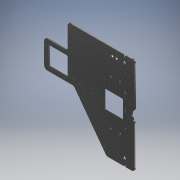
# Autodesk Inventor part: CAR SIDE PLATE I
Saved by Autodesk Inventor 2017 (Build 210142000, 142)
## iProperties
Part Number: CAR SIDE PLATE I
Material: Genérico
Document SubType Name: Modeling
Designer: Cristian
Density: 1 g/cm^3
Appearance: Valor por defecto
Author: Cristian
Autodesk Inventor part; units mm, degrees
ref_plane "YZ Plane" through (0, 0, 0) normal (1, 0, 0) x (0, 1, 0)
ref_plane "XZ Plane" through (0, 0, 0) normal (0, 1, 0) x (-1, 0, 0)
ref_plane "XY Plane" through (0, 0, 0) normal (0, 0, 1) x (1, 0, 0)
sketch "Boceto1" plane through (0, 0, 0) normal (0, 1, 0) x (-1, 0, 0)
  line L0 (0, 0) -> (273.05, 0)
  line L1 (273.05, 0) -> (273.05, -101.6)
  line L2 (273.05, -101.6) -> (368.3, -101.6)
  line L3 (368.3, -101.6) -> (368.3, -212.725)
  line L4 (0, 0) -> (0, -393.7)
  line L5 (0, -393.7) -> (114.3, -393.7)
  line L6 (368.3, -212.725) -> (247.65, -212.725)
  line L7 (247.65, -212.725) -> (114.3, -393.7)
  dimension "d0" = 273.05
  dimension "d1" = 101.6
  dimension "d2" = 95.25
  dimension "d3" = 111.125
  dimension "d4" = 393.7
  dimension "d50" = 114.3
  dimension "d51" = 133.35
  constraints: 16 end point, 3 horizontal, 2 perpendicular, 2 vertical
  measures "d0" distance of L0.start L0.end
  measures "d1" distance of L0.end L1.end
  measures "d2" distance of L1.end L2.end
  measures "d3" distance of L2.end L3.end
  measures "d4" distance of L0.start L4.end
  measures "d50" distance of L4.end L5.end
  measures "d51" horizontal distance of L5.end L6.end
extrude "Extrusión1" add sketch "Boceto1" along normal blind 5
fillet "Empalme1" radius 12.7 7 edges at (-368.3, 2.5, -101.6) (-273.05, 2.5, 0) (-368.3, 2.5, -212.725) (-247.65, 2.5, -212.725) (-114.3, 2.5, -393.7) (0, 2.5, -393.7) (0, 2.5, 0)
fillet "Empalme2" radius 6.35 1 edges at (-273.05, 2.5, -101.6)
sketch "Boceto2" plane through (0, 5, 0) normal (0, 1, 0) x (1, 0, 0)
  line L0 (-349.25, 119.0625) -> (-273.05, 119.0625)
  line L1 (-273.05, 119.0625) -> (-273.05, 195.2625)
  line L2 (-273.05, 195.2625) -> (-349.25, 195.2625)
  line L3 (-349.25, 195.2625) -> (-349.25, 119.0625)
  line L4 (-368.3, 200.025) -> (-368.3, 114.3) projected
  line L5 (-254.0674, 212.725) -> (-355.6, 212.725) projected
  line L6 (-355.6, 101.6) -> (-279.4, 101.6) projected
  line L7 (-260.35, 0) -> (-12.7, 0) projected
  line L8 (-43.6563, 0) -> (-38.1, 0)
  line L9 (-38.1, 0) -> (-38.1, 6.35)
  line L10 (-38.1, 6.35) -> (-43.6562, 6.35)
  line L11 (-43.6562, 6.35) -> (-43.6563, 0)
  line L12 (-12.7, 393.7) -> (-107.8826, 393.7) projected
  line L13 (0, 12.7) -> (0, 381) projected
  circle A0 centre (-98.0281, 104.775) radius 4.3656
  circle A1 centre (-59.9281, 104.775) radius 4.3656
  circle A2 centre (-98.0281, 288.925) radius 4.3656
  circle A3 centre (-59.9281, 288.925) radius 4.3656
  line L14 (-123.825, 158.75) -> (-47.625, 158.75)
  line L15 (-47.625, 158.75) -> (-47.625, 234.95)
  line L16 (-47.625, 234.95) -> (-123.825, 234.95)
  line L17 (-123.825, 234.95) -> (-123.825, 158.75)
  circle A4 centre (-42.6641, 365.125) radius 6.35
  circle A5 centre (-42.6641, 28.575) radius 6.35
  line L18 (-107.8826, 393.7) -> (-12.7, 393.7) projected
  line L19 (-43.6563, 393.7) -> (-38.1, 393.7)
  line L20 (-38.1, 393.7) -> (-38.1, 387.35)
  line L21 (-38.1, 387.35) -> (-43.6563, 387.35)
  line L22 (-43.6563, 387.35) -> (-43.6563, 393.7)
  line L23 (-43.6563, 127) -> (-38.1, 127)
  line L24 (-38.1, 127) -> (-38.1, 140.0969)
  line L25 (-38.1, 140.0969) -> (-43.6563, 140.0969)
  line L26 (-43.6563, 140.0969) -> (-43.6563, 127)
  line L27 (-43.6563, 190.5) -> (-38.1, 190.5)
  line L28 (-38.1, 190.5) -> (-38.1, 203.5969)
  line L29 (-38.1, 203.5969) -> (-43.6563, 203.5969)
  line L30 (-43.6563, 203.5969) -> (-43.6563, 190.5)
  line L31 (-43.6563, 254) -> (-38.1, 254)
  line L32 (-38.1, 254) -> (-38.1, 267.0969)
  line L33 (-38.1, 267.0969) -> (-43.6563, 267.0969)
  line L34 (-43.6563, 267.0969) -> (-43.6563, 254)
  circle A6 centre (-73.025, 29.3688) radius 3.9687
  circle A7 centre (-90.4875, 29.3688) radius 3.9688
  point P0 (0, 0)
  dimension "d11" = 76.2
  dimension "d17" = 17.4625
  dimension "d18" = 19.05
  dimension "d19" = 76.2
  dimension "d20" = 5.5563
  dimension "d22" = 6.35
  dimension "d24" = 38.1
  dimension "d27" = 8.7312
  dimension "d38" = 76.2
  dimension "d39" = 76.2
  dimension "d40" = 158.75
  dimension "d42" = 12.7
  dimension "d43" = 28.575
  dimension "d44" = 42.6641
  dimension "d47" = 12.7
  dimension "d52" = 38.1
  dimension "d53" = 5.5563
  dimension "d54" = 6.35
  dimension "d55" = 47.625
  dimension "d56" = 8.7312
  dimension "d57" = 98.0281
  dimension "d58" = 38.1
  dimension "d59" = 53.975
  dimension "d60" = 53.975
  dimension "d61" = 184.15
  dimension "d62" = 184.15
  dimension "d63" = 38.1
  dimension "d64" = 8.7312
  dimension "d65" = 8.7312
  dimension "d66" = 98.0281
  dimension "d67" = 42.6641
  dimension "d68" = 28.575
  dimension "d69" = 5.5563
  dimension "d70" = 5.5563
  dimension "d71" = 5.5563
  dimension "d72" = 13.0969
  dimension "d73" = 13.0969
  dimension "d74" = 13.0969
  dimension "d75" = 38.1
  dimension "d80" = 63.5
  dimension "d81" = 63.5
  dimension "d82" = 127
  dimension "d92" = 7.9375
  dimension "d93" = 7.9375
  dimension "d94" = 25.4
  dimension "d96" = 25.4
  dimension "d97" = 25.4
  dimension "d98" = 25.4
  constraints: 56 end point, 14 parallel, 8 centre point, 7 horizontal, 7 perpendicular, 3 point on line, 1 collinear
  measures "d11" distance of L2.end L0.start
  measures "d17" distance between parallel lines of L0 L6
  measures "d18" distance between parallel lines of L3 L4
  measures "d19" distance of L1.end L2.end
  measures "d20" distance between parallel lines of L9 L11
  measures "d22" distance of L10.end L8.start
  measures "d24" distance between parallel lines of L13 L9
  measures "d27" diameter of A1
  measures "d38" distance of L16.end L14.start
  measures "d39" distance between parallel lines of L15 L17
  measures "d40" distance between parallel lines of L7 L14
  measures "d42" diameter of A4
  measures "d43" distance from line of L12 A4.centre
  measures "d44" distance from line of L13 A4.centre
  measures "d47" diameter of A5
  measures "d52" distance between parallel lines of L13 L20
  measures "d53" distance between parallel lines of L20 L22
  measures "d54" distance of L21.end L19.start
  measures "d55" distance between parallel lines of L13 L15
  measures "d56" diameter of A0
  measures "d57" distance from line of L13 A0.centre
  measures "d58" distance of A1.centre A0.centre
  measures "d59" distance from line of L14 A0.centre
  measures "d60" distance from line of L14 A1.centre
  measures "d61" distance of A2.centre A0.centre
  measures "d62" distance of A1.centre A3.centre
  measures "d63" distance of A3.centre A2.centre
  measures "d64" diameter of A2
  measures "d65" diameter of A3
  measures "d66" distance from line of L13 A2.centre
  measures "d67" distance from line of L13 A5.centre
  measures "d68" distance from line of L7 A5.centre
  measures "d69" distance of L25.end L24.end
  measures "d70" distance of L29.end L28.end
  measures "d71" distance between parallel lines of L32 L34
  measures "d72" distance between parallel lines of L25 L23
  measures "d73" distance of L27.end L28.end
  measures "d74" distance of L31.end L32.end
  measures "d75" distance between parallel lines of L13 L24
  measures "d80" distance between parallel lines of L27 L23
  measures "d81" distance between parallel lines of L31 L27
  measures "d82" distance between parallel lines of L7 L23
  measures "d92" diameter of A6
  measures "d93" diameter of A7
  measures "d94" distance edge to line of A6 L11
  measures "d96" distance edge to line of A6 L7
  measures "d97" distance edge to line of A7 L7
extrude "Extrusión2" cut sketch "Boceto2" against normal up to next
fillet "Empalme3" radius 3.5719 8 edges at (-349.25, 2.5, -119.0625) (-123.825, 2.5, -158.75) (-349.25, 2.5, -195.2625) (-123.825, 2.5, -234.95) (-273.05, 2.5, -195.2625) (-47.625, 2.5, -234.95) (-273.05, 2.5, -119.0625) (-47.625, 2.5, -158.75)
sketch "Boceto3" plane through (0, 5, 0) normal (0, 1, 0) x (1, 0, 0)
  line L0 (0, 12.7) -> (0, 381) projected
  line L1 (0, 381) -> (0, 12.7) projected
  line L2 (0, 196.85) -> (-12.7, 196.85)
  line L3 (0, 196.85) -> (0, 219.075)
  line L4 (0, 196.85) -> (0, 174.625)
  arc A0 (0, 219.075) -> (0, 174.625) centre (13.0969, 196.85) ccw
  point P0 (0, 0)
  dimension "d86" = 12.7
  dimension "d87" = 22.225
  dimension "d88" = 22.225
  constraints: 6 end point, 3 point on circle, 2 point on line, 1 centre point, 1 horizontal, 1 midpoint
  measures "d86" distance of L2.start L2.end
  measures "d87" distance of L2.start L3.end
  measures "d88" distance of L2.start L4.end
extrude "Extrusión3" cut sketch "Boceto3" against normal up to next
fillet "Empalme4" radius 4.7625 2 edges at (0, 2.5, -219.075) (0, 2.5, -174.625)
equation "\"d42\" = UBD"
equation "\"d47\" = UBD"
equation "\"LM\" = 76.2"
equation "\"UBD\" = 12.7"
